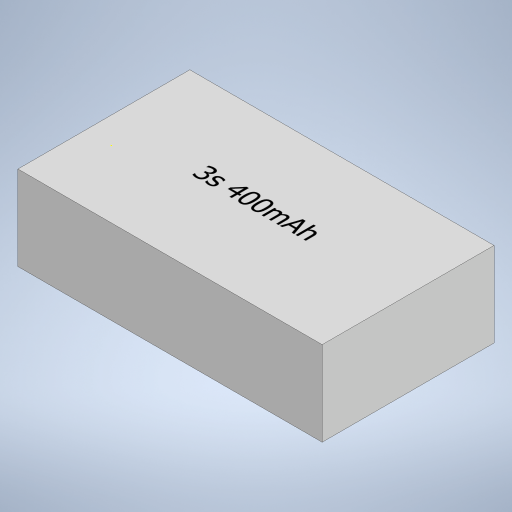
# Autodesk Inventor part: li_po3s_400mAh
Saved by Autodesk Inventor 2023 (Build 270158000, 158)
## iProperties
Created: 2025-03-19
Part Number: li_po3s_400mAh
Material: Ogólny
Document SubType Name: Modeling
Designer: kamil
Density: 1 g/cm^3
Appearance: Domyślna
Author: kamil
Autodesk Inventor part; units mm, degrees
ref_plane "YZ Plane" through (0, 0, 0) normal (1, 0, 0) x (0, 1, 0)
ref_plane "XZ Plane" through (0, 0, 0) normal (0, 1, 0) x (-1, 0, 0)
ref_plane "XY Plane" through (0, 0, 0) normal (0, 0, 1) x (1, 0, 0)
sketch "Szkic1" plane through (0, 0, 0) normal (0, 1, 0) x (-1, 0, 0)
  line L0 (4.6678, 11.8796) -> (-49.3322, 11.8796)
  line L1 (-49.3322, 11.8796) -> (-49.3322, -18.6204)
  line L2 (-49.3322, -18.6204) -> (4.6678, -18.6204)
  line L3 (4.6678, -18.6204) -> (4.6678, 11.8796)
  point P0 (0, 0)
  dimension "d0" = 54
  dimension "d1" = 30.5
  constraints: 8 end point, 2 parallel, 1 horizontal, 1 perpendicular
  measures "d0" distance of L2.end L1.end
  measures "d1" distance of L1.end L0.end
extrude "Wyciągnięcie proste1" add sketch "Szkic1" along normal blind 15
sketch "Szkic2" plane through (0, 15, 0) normal (0, 1, 0) x (1, 0, 0)
  line L0 (9.9953, 13.2196) -> (33.64, 13.2196) construction
  line L1 (33.64, 13.2196) -> (33.64, -4.8364) construction
  line L2 (33.64, -4.8364) -> (9.9953, -4.8364) construction
  line L3 (9.9953, -4.8364) -> (9.9953, 13.2196) construction
  point P0 (0, 0)
  constraints: 2 other
